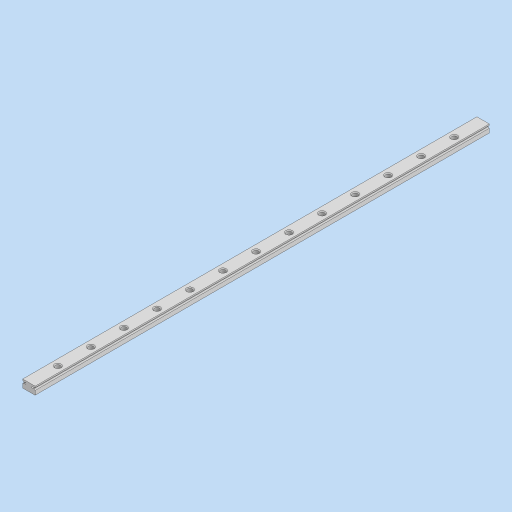
# Autodesk Inventor part: MGN15 Linear Rail 550mm
Saved by Autodesk Inventor 2023.2 (Build 272271000, 271)
## iProperties
Created: 2023-11-21
Part Number: MGN15 Linear Rail 550mm
Material: Generisch
Document SubType Name: Modeling
Designer: Nils Bade
Density: 1 g/cm^3
Appearance: Vorgabe
Author: Nils Bade
Autodesk Inventor part; units mm, degrees
ref_plane "YZ Plane" through (0, 0, 0) normal (1, 0, 0) x (0, 1, 0)
ref_plane "XZ Plane" through (0, 0, 0) normal (0, 1, 0) x (-1, 0, 0)
ref_plane "XY Plane" through (0, 0, 0) normal (0, 0, 1) x (1, 0, 0)
sketch "Skizze1" plane through (0, 0, 0) normal (0, 0, 1) x (1, 0, 0)
  line L0 (0, -1.9) -> (0, 11.4) construction
  line L1 (-7.5, 0) -> (7.5, 0)
  line L2 (7.5, 0) -> (7.5, 9.5)
  line L3 (7.5, 9.5) -> (-7.5, 9.5)
  line L4 (-7.5, 9.5) -> (-7.5, 0)
  circle A0 centre (-7.5, 6.5) radius 1.5
  line L5 (-12.6, 0) -> (12.6, 0) projected
  line L6 (-4.5, 6.5) -> (-7.5, 6.5) construction
  line L7 (-4.5, 7) -> (-7.5, 7)
  line L8 (-7.5, 6) -> (-4.5, 6)
  arc A1 (-4.5, 6) -> (-4.5, 7) centre (-4.5, 6.5) ccw
  arc A2 (-7.5, 7) -> (-7.5, 6) centre (-7.5, 6.5) ccw
  circle A3 centre (-4.5, 6.5) radius 1
  circle A4 centre (7.5, 6.5) radius 1.5
  line L9 (4.5, 7) -> (7.5, 7)
  line L10 (7.5, 6) -> (4.5, 6)
  arc A5 (4.5, 7) -> (4.5, 6) centre (4.5, 6.5) ccw
  circle A6 centre (4.5, 6.5) radius 1
  point P0 (0, 0)
  point P1 (0, 0)
  point P2 (-7.5, 8)
  point P3 (-7.5, 5)
  point P4 (-6, 6.5)
  point P5 (6, 6.5)
  point P6 (-6.0858, 7)
  point P7 (-5.366, 7)
  point P8 (-5.366, 6)
  point P9 (-6.0858, 6)
  point P10 (7.5, 5)
  point P11 (6.0858, 6)
  point P12 (5.366, 6)
  point P13 (5.366, 7)
  point P14 (6.0858, 7)
  point P15 (7.5, 8)
  dimension "d2" = 3
  dimension "d0" = 15
  dimension "d1" = 9.5
  dimension "d3" = 3
  dimension "d6" = 1
  dimension "d7" = 2
  constraints: 20 end point, 8 symmetric about line, 6 point on circle, 5 centre point, 4 tangent, 3 parallel, 2 coincident, 2 midpoint, 2 perpendicular, 2 point on line, 1 collinear, 1 horizontal, 1 vertical, 8 other
  measures "d0" distance of L1.start L1.end
  measures "d1" distance of L3.end L1.start
  measures "d3" distance from line of L6.end L3
  measures "d6" diameter of A2
  measures "d7" diameter of A3
extrude "Extrusion1" add sketch "Skizze1" along normal blind 550 contours L4 A0 L8 A3 L7 L3 L2 A4 L9 A6 L10 L1
sketch "Skizze2" plane through (-7.5, 9.5, 550) normal (0, 1, 0) x (1, 0, 0)
  line L0 (-3, 550) -> (18, 550) projected
  line L1 (7.5, 660) -> (7.5, -110) projected
  circle A0 centre (7.5, 515) radius 3
  circle A1 centre (7.5, 515) radius 1.75
  point P0 (7.5, 550)
  dimension "d8" = 6
  dimension "d9" = 3.5
  dimension "d10" = 35
  constraints: 2 centre point, 1 coincident, 1 point on line
  measures "d8" diameter of A0
  measures "d9" diameter of A1
  measures "d10" distance from line of L0 A0.centre
extrude "Extrusion2" cut sketch "Skizze2" against normal blind 6
extrude "Extrusion3" cut sketch "Skizze2" against normal blind 15 contours A1 L1 | L1 A1
chamfer "Fase1" distance 1 angle 45 1 edges at (-3, 9.5, 35)
pattern_linear "Rechteckige Anordnung1" count 13 spacing 40 along (0, 0, 1) of "Extrusion2", "Extrusion3", "Fase1"
equation "\"d4\" = Raillänge"
equation "\"Raillänge\" = 550"
